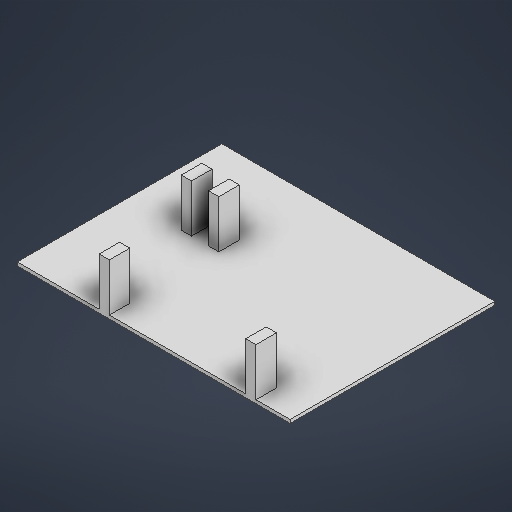
# Autodesk Inventor part: base
Saved by Autodesk Inventor 2026.1 (Build 301233020, 233B)
## iProperties
Created: 2025-12-30
Part Number: base
Material: Generic
Document SubType Name: Modeling
Designer: Austin Ngobeni
Density: 1 g/cm^3
Appearance: Default
clampwidth: 30.000 mm
clampheight: 60.000 mm
d36: 60.000 mm
d37: 30.000 mm
Author: Austin Ngobeni
Autodesk Inventor part; units mm, degrees
ref_plane "YZ Plane" through (0, 0, 0) normal (1, 0, 0) x (0, 1, 0)
ref_plane "XZ Plane" through (0, 0, 0) normal (0, 1, 0) x (-1, 0, 0)
ref_plane "XY Plane" through (0, 0, 0) normal (0, 0, 1) x (1, 0, 0)
sketch "Sketch1" plane through (0, 0, 0) normal (0, 1, 0) x (-1, 0, 0)
  line L0 (350, -300) -> (-450, -300)
  line L1 (-450, -300) -> (-450, 300)
  line L2 (-450, 300) -> (350, 300)
  line L3 (350, 300) -> (350, -300)
  line L4 (-450, 240) -> (-450, 300)
  line L5 (110, 300) -> (80, 300)
  line L6 (80, 300) -> (80, 240)
  line L7 (80, 240) -> (110, 240)
  line L8 (110, 240) -> (110, 300)
  line L9 (110, -81.09) -> (80, -81.09)
  line L10 (80, -81.09) -> (80, -21.09)
  line L11 (80, -21.09) -> (110, -21.09)
  line L12 (110, -21.09) -> (110, -81.09)
  line L13 (-320, 300) -> (-350, 300)
  line L14 (-350, 300) -> (-350, 240)
  line L15 (-350, 240) -> (-320, 240)
  line L16 (-320, 240) -> (-320, 300)
  line L17 (190, -81.09) -> (160, -81.09)
  line L18 (160, -81.09) -> (160, -21.09)
  line L19 (160, -21.09) -> (190, -21.09)
  line L20 (190, -21.09) -> (190, -81.09)
  point P0 (-50, 300)
  point P1 (350, 0)
  point P2 (95, 240)
  point P3 (80, 300)
  point P4 (110, -51.09)
  point P5 (110, 270)
  point P6 (-350, 300)
  point P7 (80, 270)
  point P8 (190, -51.09)
  dimension "d0" = 600
  dimension "d1" = 800
  dimension "d22" = 60
  dimension "d23" = 30
  dimension "d27" = 321.09
  dimension "d28" = 30
  dimension "d31" = 400
  dimension "d32" = 60
  dimension "d33" = 30
  dimension "d38" = 50
  constraints: 42 end point, 11 parallel, 7 midpoint, 5 horizontal, 5 perpendicular, 2 point on line, 1 vertical, 1 vertical alignment, 1 other
  measures "d0" distance of L2.end L0.start
  measures "d1" distance of L0.start L0.end
  measures "d22" distance of L11.end L9.start
  measures "d23" distance of L9.start L9.end
  measures "d27" distance of point (110, -51.09) point (110, 270)
  measures "d28" distance of L14.end L15.end
  measures "d31" distance between parallel lines of L16 L6
  measures "d32" distance of L19.end L17.start
  measures "d33" distance of L17.start L18.start
  measures "d38" distance between parallel lines of L12 L18
extrude "Extrusion1" add sketch "Sketch1" along normal blind 10 contours L0 L1 L2 L14 L15 L16 L6 L7 L8 L3 | L2 L16 L15 L14 | L9 L10 L11 L12 | L17 L18 L19 L20
extrude "Extrusion6" add sketch "Sketch1" along normal blind 150 contours L9 L10 L11 L12
extrude "Extrusion7" add sketch "Sketch1" along normal blind 150 contours L8 L7 L6 L2 | L2 L16 L15 L14
extrude "Extrusion8" add sketch "Sketch1" along normal blind 150 contours L17 L18 L19 L20
equation "\"d22\" = d3"
equation "\"d23\" = d2"
equation "\"d28\" = d23"
equation "\"d32\" = d34"
equation "\"d33\" = d35"
equation "\"d3\" = 60"
equation "\"d2\" = 30"
equation "\"d34\" = 60"
equation "\"d35\" = 30"
body "Solid1"
